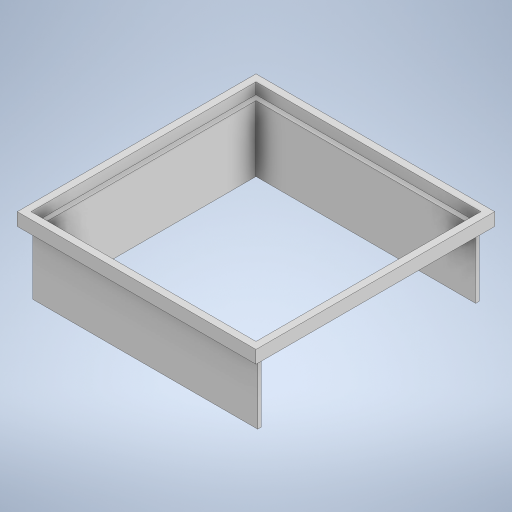
# Autodesk Inventor part: wall support
Saved by Autodesk Inventor 2024 (Build 280153000, 153)
## iProperties
Created: 2024-04-18
Part Number: wall support
Material: Generic
Document SubType Name: Modeling
Designer: drew
Density: 1 g/cm^3
Appearance: Default
Author: drew
Autodesk Inventor part; units mm, degrees
ref_plane "YZ Plane" through (0, 0, 0) normal (1, 0, 0) x (0, 1, 0)
ref_plane "XZ Plane" through (0, 0, 0) normal (0, 1, 0) x (-1, 0, 0)
sketch "Sketch1" plane through (0, 0, 0) normal (0, 1, 0) x (-1, 0, 0)
  line L0 (-103.1875, 101.6) -> (103.1875, 101.6)
  line L1 (103.1875, 101.6) -> (103.1875, -101.6)
  line L2 (103.1875, -101.6) -> (-103.1875, -101.6)
  line L3 (-103.1875, -101.6) -> (-103.1875, 101.6)
  line L4 (-103.1875, 101.6) -> (103.1875, -101.6) construction
  line L5 (103.1875, 101.6) -> (-103.1875, -101.6) construction
  line L6 (-98.425, 98.425) -> (98.425, 98.425)
  line L7 (98.425, 98.425) -> (98.425, -98.425)
  line L8 (98.425, -98.425) -> (-98.425, -98.425)
  line L9 (-98.425, -98.425) -> (-98.425, 98.425)
  line L10 (-98.425, 98.425) -> (98.425, -98.425) construction
  line L11 (98.425, 98.425) -> (-98.425, -98.425) construction
  point P0 (0, 0)
  dimension "d0" = 203.2
  dimension "d1" = 206.375
  dimension "d2" = 196.85
  constraints: 24 end point, 4 midpoint, 4 parallel, 3 perpendicular, 2 horizontal
  measures "d0" distance of L0.end L1.end
  measures "d1" distance of L1.end L2.end
  measures "d2" distance of L6.end L7.end
extrude "Extrusion1" add sketch "Sketch1" along normal blind 60.325
ref_plane "Work Plane1" through (0, 58.7375, 0) normal (0, 1, 0) x (1, 0, 0)
sketch "Sketch2" plane through (0, 58.7375, 0) normal (0, 1, 0) x (1, 0, 0)
  line L0 (109.5375, -109.5375) -> (-109.5375, -109.5375)
  line L1 (-109.5375, -109.5375) -> (-109.5375, 109.5375)
  line L2 (-109.5375, 109.5375) -> (109.5375, 109.5375)
  line L3 (109.5375, 109.5375) -> (109.5375, -109.5375)
  line L4 (109.5375, -109.5375) -> (-109.5375, 109.5375) construction
  line L5 (-109.5375, -109.5375) -> (109.5375, 109.5375) construction
  line L6 (103.1875, 101.6) -> (-103.1875, 101.6) projected
  line L7 (-103.1875, 101.6) -> (-103.1875, -101.6) projected
  line L8 (-103.1875, -101.6) -> (103.1875, -101.6) projected
  line L9 (103.1875, -101.6) -> (103.1875, 101.6) projected
  line L10 (98.425, -98.425) -> (-98.425, -98.425) projected
  line L11 (-98.425, -98.425) -> (-98.425, 98.425) projected
  line L12 (-98.425, 98.425) -> (98.425, 98.425) projected
  line L13 (98.425, 98.425) -> (98.425, -98.425) projected
  point P0 (0, 0)
  dimension "d7" = 219.075
  constraints: 12 end point, 2 midpoint, 2 parallel, 2 perpendicular, 1 horizontal
  measures "d7" distance of L1.end L2.end
extrude "Extrusion2" add sketch "Sketch2" along normal up to surface (1.5875 mm away) contours L0 L1 L2 L3
sketch "Sketch3" plane through (0, 60.325, 0) normal (0, 1, 0) x (1, 0, 0)
  line L0 (109.5375, 109.5375) -> (109.5375, -109.5375) projected
  line L1 (-109.5375, 109.5375) -> (109.5375, 109.5375) projected
  line L2 (-109.5375, -109.5375) -> (-109.5375, 109.5375) projected
  line L3 (109.5375, -109.5375) -> (-109.5375, -109.5375) projected
  line L4 (98.425, -98.425) -> (-98.425, -98.425) projected
  line L5 (-98.425, -98.425) -> (-98.425, 98.425) projected
  line L6 (-98.425, 98.425) -> (98.425, 98.425) projected
  line L7 (98.425, 98.425) -> (98.425, -98.425) projected
  line L8 (103.1875, -103.1875) -> (-103.1875, -103.1875)
  line L9 (-103.1875, -103.1875) -> (-103.1875, 103.1875)
  line L10 (-103.1875, 103.1875) -> (103.1875, 103.1875)
  line L11 (103.1875, 103.1875) -> (103.1875, -103.1875)
  line L12 (103.1875, -103.1875) -> (-103.1875, 103.1875) construction
  line L13 (-103.1875, -103.1875) -> (103.1875, 103.1875) construction
  point P0 (0, 0)
  dimension "d10" = 206.375
  constraints: 12 end point, 2 midpoint, 2 parallel, 2 perpendicular, 1 horizontal
  measures "d10" distance of L9.end L10.end
extrude "Extrusion3" add sketch "Sketch3" along normal blind 10.16 contours L0 L3 L2 L1
sketch "Sketch4" plane through (103.1875, 0, 101.6) normal (1, 0, 0) x (0, 0, -1)
  line L0 (200.025, 0) -> (3.175, 0) projected
  line L1 (3.175, 0) -> (3.175, 60.325) projected
  line L2 (200.025, 60.325) -> (3.175, 60.325) projected
  line L3 (200.025, 0) -> (200.025, 60.325) projected
  point P0 (101.6, 0)
extrude "Extrusion4" cut sketch "Sketch4" against normal blind 10.16
body "Solid1"
